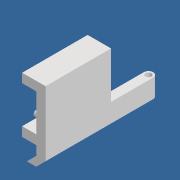
# Autodesk Inventor part: MotorHolder_X_R
Saved by Autodesk Inventor 2020 (Build 240168000, 168)
## iProperties
Created: 2019-12-21
Part Number: MotorHolder_X_R
Material: Generic
Document SubType Name: Modeling
Designer: Jack
Density: 1 g/cm^3
Appearance: Default
Author: Jack
Autodesk Inventor part; units mm, degrees
ref_plane "YZ Plane" through (0, 0, 0) normal (1, 0, 0) x (0, 1, 0)
ref_plane "XZ Plane" through (0, 0, 0) normal (0, 1, 0) x (-1, 0, 0)
ref_plane "XY Plane" through (0, 0, 0) normal (0, 0, 1) x (1, 0, 0)
sketch "Sketch1" plane through (0, 0, 0) normal (1, 0, 0) x (0, 1, 0)
  line L0 (-19.8, 28) -> (19.8, 28)
  line L1 (19.8, 28) -> (19.8, -28)
  line L2 (19.8, -28) -> (-19.8, -28)
  line L3 (-19.8, -28) -> (-19.8, 28)
  line L4 (-19.8, 28) -> (19.8, -28) construction
  line L5 (19.8, 28) -> (-19.8, -28) construction
  point P0 (0, 0)
  dimension "d0" = 39.6
  dimension "d1" = 56
  constraints: 12 end point, 2 midpoint, 2 parallel, 1 horizontal, 1 perpendicular
  measures "d0" distance of L1.end L2.end
  measures "d1" distance of L0.end L1.end
extrude "Extrusion1" add sketch "Sketch1" along normal blind 40
sketch "Sketch2" plane through (0, -19.8, 28) normal (0, 0, 1) x (1, 0, 0)
  line L0 (7.8, 0) -> (32.2, 0)
  line L1 (32.2, 0) -> (32.2, 31.8)
  line L2 (32.2, 31.8) -> (7.8, 31.8)
  line L3 (7.8, 31.8) -> (7.8, 0)
  line L4 (0, 0) -> (40, 0) projected
  line L5 (40, 39.6) -> (40, 0) projected
  dimension "d4" = 24.4
  dimension "d5" = 31.8
  dimension "d6" = 7.8
  constraints: 8 end point, 2 parallel, 1 horizontal, 1 perpendicular, 1 point on line
  measures "d4" distance of L2.end L1.end
  measures "d5" distance of L1.end L0.end
  measures "d6" distance between parallel lines of L5 L1
extrude "Extrusion2" cut sketch "Sketch2" against normal blind 64
sketch "Sketch3" plane through (32.2, -19.8, 28) normal (-1, 0, 0) x (0, 0, 1)
  circle A0 centre (-12, 3.8502) radius 2.3
  circle A1 centre (-28, 3.8502) radius 2.3
  line L0 (0, 31.8) -> (0, 0) projected
  point P0 (-28, 19.8)
  dimension "d9" = 4.6
  dimension "d10" = 4.6
  dimension "d11" = 16
  dimension "d12" = 12
  constraints: 2 centre point, 1 horizontal alignment
  measures "d9" diameter of A0
  measures "d10" diameter of A1
  measures "d11" distance of A1.centre A0.centre
  measures "d12" distance from line of L0 A0.centre
extrude "Extrusion3" add sketch "Sketch3" along normal blind 26
sketch "Sketch4" plane through (7.8, -19.8, 28) normal (1, 0, 0) x (0, 0, -1)
  line L0 (56, 0) -> (0, 0) projected
  line L1 (56, 0) -> (32, 0)
  line L2 (32, 0) -> (32, 8)
  line L3 (32, 8) -> (56, 8)
  line L4 (56, 8) -> (56, 0)
  point P0 (28, 19.8)
  point P1 (32, 0)
  dimension "d15" = 24
  dimension "d16" = 8
  constraints: 8 end point, 2 parallel, 1 horizontal, 1 perpendicular
  measures "d15" distance of L2.end L3.end
  measures "d16" distance of L1.end L2.end
extrude "Extrusion4" add sketch "Sketch4" along normal blind 26
sketch "Sketch14" plane through (0, 19.8, 28) normal (0, 1, 0) x (1, 0, 0)
  line L0 (20, 0) -> (20, 56) projected
  point P0 (0, 28)
sketch "Sketch15" plane through (0, -19.8, -28) normal (0, -1, 0) x (1, 0, 0)
  line L0 (40, 0) -> (40, 56) projected
  line L1 (0, 0) -> (40, 0) projected
  line L2 (0, 56) -> (40, 56) projected
  line L3 (0, 0) -> (0, 56) projected
  point P0 (0, 28)
extrude "Extrusion7" add sketch "Sketch15" along normal blind 24
sketch "Sketch16" plane through (0, 19.8, 28) normal (0, 0, 1) x (1, 0, 0)
  line L0 (8, -47.6) -> (32, -47.6)
  line L1 (32, -47.6) -> (32, -55.6)
  line L2 (32, -55.6) -> (8, -55.6)
  line L3 (8, -55.6) -> (8, -47.6)
  line L4 (40, -63.6) -> (0, -63.6) projected
  line L5 (0, 0) -> (0, -63.6) projected
  line L6 (16, -55.6) -> (24, -55.6)
  line L7 (24, -55.6) -> (24, -63.6)
  line L8 (24, -63.6) -> (16, -63.6)
  line L9 (16, -63.6) -> (16, -55.6)
  point P0 (0, -19.8)
  dimension "d37" = 24
  dimension "d38" = 8
  dimension "d39" = 8
  dimension "d40" = 8
  dimension "d41" = 8
  dimension "d42" = 8
  dimension "d43" = 16
  constraints: 16 end point, 4 parallel, 2 horizontal, 2 perpendicular, 1 point on line
  measures "d37" distance of L1.end L2.end
  measures "d38" distance of L0.end L1.end
  measures "d39" distance between parallel lines of L4 L2
  measures "d40" distance between parallel lines of L5 L3
  measures "d41" distance of L7.end L8.end
  measures "d42" distance of L6.end L7.end
  measures "d43" distance between parallel lines of L5 L9
extrude "Extrusion8" cut sketch "Sketch16" against normal through all
chamfer "Chamfer1" distance 8 angle 45 2 edges at (40, -43.8, 0) (0, -43.8, 0)
chamfer "Chamfer2" distance 8 angle 45 2 edges at (16, -35.8, 0) (24, -35.8, 0)
split body "Split2" sketch "Sketch14" result one side removed curves L0 removed pieces at (0.5, -17.2667, 9.3333)
sketch "Sketch17" plane through (20, -27.8, -28) normal (-1, 0, 0) x (0, 0, 1)
  circle A0 centre (12, 3.6) radius 2.5
  circle A1 centre (28, 3.6) radius 2.5
  circle A2 centre (44, 3.6) radius 2.5
  circle A3 centre (12, 43.6) radius 2.5
  circle A4 centre (44, 43.6) radius 2.5
  circle A5 centre (28, 43.6) radius 2.5
  line L0 (0, 47.6) -> (56, 47.6) projected
  line L1 (0, 39.8) -> (0, 47.6) projected
  point P0 (28, 27.8)
  dimension "d52" = 5
  dimension "d53" = 5
  dimension "d55" = 5
  dimension "d56" = 5
  dimension "d57" = 5
  dimension "d58" = 5
  dimension "d59" = 16
  dimension "d60" = 16
  dimension "d61" = 40
  dimension "d62" = 4
  dimension "d63" = 12
  constraints: 6 centre point, 4 horizontal alignment, 3 vertical alignment
  measures "d52" diameter of A0
  measures "d53" diameter of A1
  measures "d55" diameter of A2
  measures "d56" diameter of A3
  measures "d57" diameter of A4
  measures "d58" diameter of A5
  measures "d59" distance of A5.centre A3.centre
  measures "d60" distance of A4.centre A5.centre
  measures "d61" distance of A0.centre A3.centre
  measures "d62" distance from line of L0 A3.centre
  measures "d63" distance from line of L1 A3.centre
extrude "Extrusion9" cut sketch "Sketch17" against normal blind 8
sketch "Sketch22" plane through (32.2, -11.8, -28) normal (0, 0, -1) x (-1, 0, 0)
  line L0 (0.2, -32) -> (-7.8, -24) projected
  line L1 (-7.8, -24) -> (0.2, -24)
  line L2 (0.2, -24) -> (0.2, -8)
  line L3 (0.2, -8) -> (-7.8, -8)
  line L4 (-7.8, -8) -> (-7.8, -24)
  point P0 (32.2, 11.8)
  dimension "d82" = 8
  dimension "d83" = 16
  constraints: 8 end point, 2 parallel, 1 horizontal, 1 perpendicular
  measures "d82" distance of L3.end L2.end
  measures "d83" distance of L2.end L1.end
extrude "Extrusion13" add sketch "Sketch22" along normal blind 40
sketch "Sketch23" plane through (32, -19.8, -28) normal (0, 1, 0) x (1, 0, 0)
  circle A0 centre (4, 36) radius 2.5
  line L0 (8, 0) -> (8, 40) projected
  line L1 (0, 40) -> (8, 40) projected
  point P0 (-32, -28)
  dimension "d86" = 5
  dimension "d87" = 4
  dimension "d88" = 4
  constraints: 1 centre point
  measures "d86" diameter of A0
  measures "d87" distance from line of L0 A0.centre
  measures "d88" distance from line of L1 A0.centre
extrude "Extrusion14" cut sketch "Sketch23" against normal through all
fillet "Fillet2" radius 4 2 edges at (40, -27.8, -68) (32, -27.8, -68)
body "Solid1"
